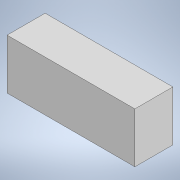
# Autodesk Inventor part: thermister
Saved by Autodesk Inventor 2022.1 (Build 261234000, 234)
## iProperties
Created: 2021-08-22
Part Number: thermister
Material: Generic
Document SubType Name: Modeling
Designer: robst
Density: 1 g/cm^3
Appearance: Default
Author: robst
Autodesk Inventor part; units mm, degrees
ref_plane "YZ Plane" through (0, 0, 0) normal (1, 0, 0) x (0, 1, 0)
ref_plane "XZ Plane" through (0, 0, 0) normal (0, 1, 0) x (-1, 0, 0)
ref_plane "XY Plane" through (0, 0, 0) normal (0, 0, 1) x (1, 0, 0)
sketch "Sketch1" plane through (0, 0, 0) normal (0, 0, 1) x (1, 0, 0)
  line L0 (-33.6, -13.2) -> (33.6, -13.2)
  line L1 (33.6, -13.2) -> (33.6, 13.2)
  line L2 (33.6, 13.2) -> (-33.6, 13.2)
  line L3 (-33.6, 13.2) -> (-33.6, -13.2)
  line L4 (-33.6, -13.2) -> (33.6, 13.2) construction
  line L5 (33.6, -13.2) -> (-33.6, 13.2) construction
  point P0 (0, 0)
  dimension "d0" = 67.2
  dimension "d1" = 26.4
  constraints: 12 end point, 2 midpoint, 2 parallel, 1 horizontal, 1 perpendicular
  measures "d0" distance of L0.start L0.end
  measures "d1" distance of L2.end L0.start
extrude "Extrusion1" add sketch "Sketch1" along normal blind 20
equation "\"d0\" = thermisterLength"
equation "\"d1\" = thermisterWidth"
equation "\"d2\" = thermisterDepth"
equation "\"thermisterWidth\" = 26.4"
equation "\"thermisterLength\" = 67.2"
equation "\"thermisterDepth\" = 20"
body "Solid1"
